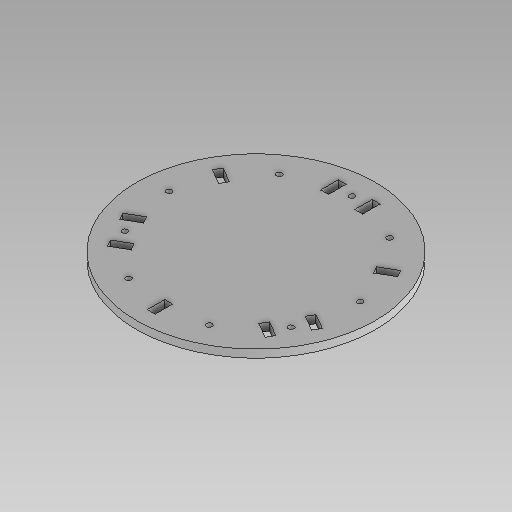
# Autodesk Inventor part: Prototype Plate Base
Saved by Autodesk Inventor 2020.1 (Build 241239000, 239)
## iProperties
Created: 2019-08-27
Part Number: Prototype Plate Base
Material: Generic
Document SubType Name: Modeling
Designer: Oliver Frolovs
Mass: 383.195 g
Surface Area: 1043.06 cm^2
Volume: 383.195 cm^3
Density: 1 g/cm^3
Appearance: Default
Author: Oliver Frolovs
Autodesk Inventor part; units mm, degrees
ref_plane "YZ Plane" through (0, 0, 0) normal (1, 0, 0) x (0, 1, 0)
ref_plane "XZ Plane" through (0, 0, 0) normal (0, 1, 0) x (-1, 0, 0)
ref_plane "XY Plane" through (0, 0, 0) normal (0, 0, 1) x (1, 0, 0)
sketch "Sketch the Prototype Plate Base Profile" plane through (0, 0, 0) normal (0, 0, 1) x (1, 0, 0)
  circle A0 centre (0, 0) radius 137
  dimension "d0" = 274
  constraints: 1 centre point, 1 coincident
  measures "d0" diameter of A0
extrude "Make Prototype Plate Base by Extrusion" add sketch "Sketch the Prototype Plate Base Profile" along normal mid plane 9
sketch "Locate the Outer Rib Slots" plane through (0, 0, 4.5) normal (0, 0, 1) x (1, 0, 0)
  circle A0 centre (0, 0) radius 137 projected
  line L0 (0, 0) -> (0, 137) construction
  circle A1 centre (0, 137) radius 15 construction
  line L1 (-24, 118.2578) -> (-15, 118.2578)
  line L2 (-15, 118.2578) -> (-15, 98.2578)
  line L3 (-15, 98.2578) -> (-24, 98.2578)
  line L4 (-24, 98.2578) -> (-24, 118.2578)
  line L5 (-24, 118.2578) -> (-15, 98.2578) construction
  line L6 (-15, 118.2578) -> (-24, 98.2578) construction
  line L7 (-19.5, 108.2578) -> (-15, 108.2578) construction
  circle A2 centre (0, 0) radius 61 construction
  line L8 (24, 118.2578) -> (15, 118.2578)
  line L9 (15, 118.2578) -> (15, 98.2578)
  line L10 (15, 98.2578) -> (24, 98.2578)
  line L11 (24, 98.2578) -> (24, 118.2578)
  circle A3 centre (0, 0) radius 110 construction
  line L12 (-15, 98.2578) -> (0, 98.2578) construction
  dimension "d29" = 220
  dimension "d3" = 30
  dimension "d5" = 20
  dimension "d15" = 9
  dimension "d17" = 122
  dimension "d30" = 15
  constraints: 26 end point, 4 symmetric about line, 3 coincident, 2 centre point, 2 horizontal, 2 midpoint, 2 perpendicular, 1 parallel, 1 point on line, 1 vertical, 1 vertical alignment, 4 other
  measures "d3" diameter of A1
  measures "d5" distance of L3.end L1.start
  measures "d15" distance of L2.end L3.end
  measures "d17" diameter of A2
  measures "d30" distance of L2.end L12.end
extrude "Cut Outer Rib Slots" cut sketch "Locate the Outer Rib Slots" against normal blind 9 contours L1 L2 L3 L4 | L11 L10 L9 L8
pattern_circular "Pattern Outer Rib Slots Around the Base Plate" count 3 over 360 about axis through (0, 0, -10) along (0, 0, 1) of "Cut Outer Rib Slots"
sketch "Locate the Inner Rib Slot" plane through (0, 0, 4.5) normal (0, 0, 1) x (1, 0, 0)
  circle A0 centre (0, 0) radius 137 projected
  line L0 (-106.173, 56.1029) -> (-101.673, 63.8971)
  line L1 (-101.673, 63.8971) -> (-84.3525, 53.8971)
  line L2 (-84.3525, 53.8971) -> (-88.8525, 46.1029)
  line L3 (-88.8525, 46.1029) -> (-106.173, 56.1029)
  line L4 (-106.173, 56.1029) -> (-84.3525, 53.8971) construction
  line L5 (-101.673, 63.8971) -> (-88.8525, 46.1029) construction
  circle A1 centre (0, 0) radius 110 construction
  line L6 (-95.2628, 55) -> (0, 0) construction
  line L7 (0, -210.7) -> (0, 210.7) projected
  dimension "d31" = 220
  dimension "d27" = 9
  dimension "d28" = 20
  dimension "d32" = 60
  constraints: 14 end point, 2 midpoint, 2 parallel, 2 perpendicular, 1 coincident, 3 other
  measures "d27" distance of L1.end L2.end
  measures "d28" distance of L0.end L1.end
  measures "d32" angle of L7 L6
extrude "Cut Inner Rib Slots" cut sketch "Locate the Inner Rib Slot" against normal blind 9 contours L0 L1 L2 L3
pattern_circular "Pattern Inner Rib Slots Around the Base Plate" count 3 over 360 about axis through (0, 0, -10) along (0, 0, 1) of "Cut Inner Rib Slots"
sketch "Locate Holes for Connecting Two Bases" plane through (0, 0, 4.5) normal (0, 0, 1) x (1, 0, 0)
  circle A0 centre (0, 0) radius 137 projected
  line L0 (-15, 118.2578) -> (-15, 98.2578) projected
  line L1 (15, 98.2578) -> (15, 118.2578) projected
  circle A1 centre (0, 0) radius 110 construction
  line L2 (0, 0) -> (0, 110) construction
  line L3 (-24, 98.2578) -> (-24, 118.2578) projected
  line L4 (-101.673, 63.8971) -> (-84.3525, 53.8971) projected
  circle A2 centre (-92.933, 58.8511) radius 42.9699 construction
  circle A3 centre (-24, 107.3499) radius 42.9699 construction
  line L5 (24, 118.2578) -> (24, 98.2578) projected
  line L6 (84.3525, 53.8971) -> (101.673, 63.8971) projected
  circle A4 centre (24, 107.3499) radius 42.9699 construction
  circle A5 centre (92.933, 58.8511) radius 42.9699 construction
  point P0 (-63.2959, 89.9646)
  point P1 (63.2959, 89.9646)
  point P2 (-46.2637, -99.7981)
  point P3 (-109.5596, 9.8335)
  point P4 (109.5596, 9.8335)
  point P5 (46.2637, -99.7981)
  dimension "d54" = 220
  dimension "d66" = 360
  constraints: 4 point on line, 2 end point, 1 coincident, 1 vertical, 28 other
hole "Clearance Holes to Bolt the Two Bases Together" at (-63.2959, 89.9646, 4.5) at (63.2959, 89.9646, 4.5) at (-46.2637, -99.7981, 4.5) at (-109.5596, 9.8335, 4.5) at (109.5596, 9.8335, 4.5) at (46.2637, -99.7981, 4.5) direction (0, 0, -1) diameter 6.4 end through all clearance for "Socket Head Cap Screw ISO 4762" size "M6" standard "ISO"
sketch3d "Locate Three More Holes to Support the Connection Between Tw"
  constraints: 2 end point, 1 coincident, 1 vertical, 1 vertical alignment, 6 other
hole "Clearance Holes to Bolt the Two Bases Together at Arms" at (0, 110, 4.5) at (-95.2628, -55, 4.5) at (95.2628, -55, 4.5) direction (0, 0, -1) diameter 6.4 end through all clearance for "Socket Head Cap Screw ISO 4762" size "M6" standard "ISO"
equation "\"d0\" = PrototypePlateDiameter"
equation "\"d1\" = PrototypePlateMaterialThickness"
equation "\"d29\" = OuterRibSlotPCD"
equation "\"d3\" = RigColumnsDiameter"
equation "\"d5\" = RibSlotLength"
equation "\"d15\" = PrototypePlateRibMaterialThickness"
equation "\"d30\" = 0.5 * RigColumnsDiameter"
equation "\"d18\" = PrototypePlateMaterialThickness"
equation "\"d31\" = InnerRibSlotPCD"
equation "\"d27\" = PrototypePlateRibMaterialThickness"
equation "\"d28\" = RibSlotLength"
equation "\"d33\" = PrototypePlateMaterialThickness"
equation "\"d54\" = InnerRibSlotPCD"
equation "\"d75\" = InnerRibSlotPCD"
equation "\"PrototypePlateDiameter\" = 274"
equation "\"PrototypePlateMaterialThickness\" = 9"
equation "\"OuterRibSlotPCD\" = 220"
equation "\"RigColumnsDiameter\" = 30"
equation "\"RibSlotLength\" = 20"
equation "\"PrototypePlateRibMaterialThickness\" = 9"
equation "\"InnerRibSlotPCD\" = 220"
body "Solid1"
